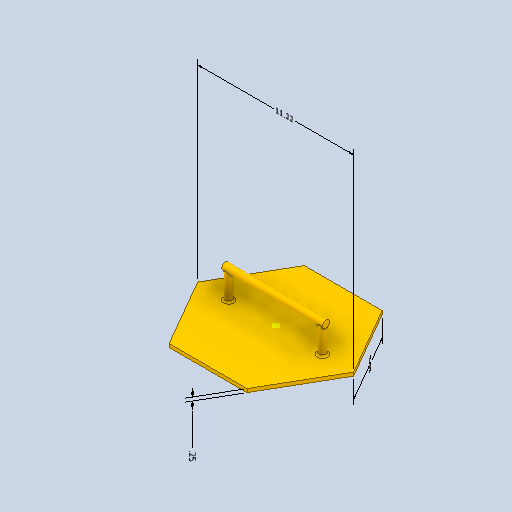
# Autodesk Inventor part: HL-01
Saved by Autodesk Inventor 2022 (Build 260153000, 153)
## iProperties
Company: El Camino College
Created: 2023-05-12
Part Number: HL-01
Material: Aluminum 6061 Painted
Document SubType Name: Modeling
Designer: Edgar Tejada
Density: 2.7 g/cm^3
Appearance: Aluminum - Flat(1)
Mass: 999.071 g
Surface Area: 1215.62 cm^2
Volume: 370.026 cm^3
Project: Hexagonal Hive
Description: Aluminum Lid with Handle
Author: Edgar Tejada
Title: Hexagonal Lid
Subject: Hexagonal Hive
Autodesk Inventor part; units mm, degrees
ref_plane "YZ Plane" through (0, 0, 0) normal (1, 0, 0) x (0, 1, 0)
ref_plane "XZ Plane" through (0, 0, 0) normal (0, 1, 0) x (-1, 0, 0)
ref_plane "XY Plane" through (0, 0, 0) normal (0, 0, 1) x (1, 0, 0)
sketch "Sketch1" plane through (0, 0, 0) normal (0, 1, 0) x (-1, 0, 0)
  circle A0 centre (0, 0) radius 95.25 construction
  circle A1 centre (0, 0) radius 120.65 construction
  line L0 (-69.6573, -120.65) -> (-139.3146, 0)
  line L1 (-139.3146, 0) -> (-69.6573, 120.65)
  line L2 (-69.6573, 120.65) -> (69.6573, 120.65)
  line L3 (69.6573, 120.65) -> (139.3146, 0)
  line L4 (139.3146, 0) -> (69.6573, -120.65)
  line L5 (69.6573, -120.65) -> (-69.6573, -120.65)
  line L6 (142.4896, 0) -> (71.2448, 123.3996)
  line L7 (71.2448, 123.3996) -> (-71.2448, 123.3996)
  line L8 (-71.2448, 123.3996) -> (-142.4896, 0)
  line L9 (-142.4896, 0) -> (-71.2448, -123.3996)
  line L10 (-71.2448, -123.3996) -> (71.2448, -123.3996)
  line L11 (71.2448, -123.3996) -> (142.4896, 0)
  dimension "d0" = 190.5
  dimension "d1" = 25.4
  dimension "d2" = 3.175
  dimension "d15" = 278.6292
  constraints: 24 end point, 3 coincident, 2 centre point, 1 horizontal alignment, 1 tangent, 18 other
  measures "d0" diameter of A0
  measures "d1" radial gap between concentric circles of A1 A0
  measures "d2" distance of L3.end L6.start
  measures "d15" distance of L0.end L3.end
extrude "Extrusion1" add sketch "Sketch1" along normal blind 6.35 contours L0 L1 L2 L3 L4 L5 | L11 L10 L9 L8 L7 L6
sketch "Sketch2" plane through (0, 6.35, 0) normal (0, 1, 0) x (1, 0, 0)
  point P0 (0, 0)
sketch "Sketch3" plane through (0, 6.35, 0) normal (0, 1, 0) x (1, 0, 0)
  circle A0 centre (-85.725, 0) radius 6.35
  circle A1 centre (85.725, 0) radius 6.35
  point P0 (0, 0)
  dimension "d16" = 12.7
  dimension "d17" = 171.45
  dimension "d18" = 85.725
  constraints: 2 centre point, 2 horizontal alignment, 1 equal radius
  measures "d16" diameter of A0
  measures "d17" distance of A1.centre A0.centre
  measures "d18" distance of point (0, 0) A1.centre
extrude "Extrusion2" add sketch "Sketch3" along normal blind 50.8
sketch "Sketch4" plane through (0, 0, 0) normal (1, 0, 0) x (0, 1, 0)
  line L0 (57.15, -6.35) -> (57.15, 6.35) projected
  circle A0 centre (57.15, 0) radius 6.35
  point P0 (0, 0)
  constraints: 1 midpoint, 1 vertical alignment, 2 other
extrude "Extrusion3" add sketch "Sketch4" along normal mid plane 184.15
fillet "Fillet2" radius 3.175 10 edges at (79.375, 6.35, 0) (90.2151, 52.6599, 4.4901) (81.2349, 52.6599, 4.4901) (81.2349, 52.6599, -4.4901) (-81.2349, 52.6599, 4.4901) (-81.2349, 52.6599, -4.4901) (-90.2151, 52.6599, -4.4901) (-92.075, 6.35, 0) (-90.2151, 52.6599, 4.4901) (90.2151, 52.6599, -4.4901)
equation "\"d18\" = 0.5 * d17"
equation "\"d21\" = d17 + 0.25 * d19"
equation "\"d19\" = 50.8"
body "Solid1"
